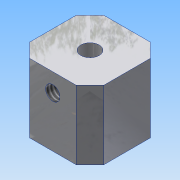
# Autodesk Inventor part: Drehmomentuebertraeger_V4_1
Saved by Autodesk Inventor 2015 (Build 190159000, 159)
## iProperties
Created: 2015-09-28
Part Number: Drehmomentuebertraeger_V4_1
Material: Aluminium 6061
Document SubType Name: Modeling
Designer: Johann
Density: 2.7 g/cm^3
Appearance: Aluminium - flach
Author: Johann
Autodesk Inventor part; units mm, degrees
ref_plane "YZ Plane" through (0, 0, 0) normal (1, 0, 0) x (0, 1, 0)
ref_plane "XZ Plane" through (0, 0, 0) normal (0, 1, 0) x (-1, 0, 0)
ref_plane "XY Plane" through (0, 0, 0) normal (0, 0, 1) x (1, 0, 0)
sketch "Skizze1" plane through (0, 0, 0) normal (0, 0, 1) x (1, 0, 0)
  line L0 (-4.05, -4.05) -> (4.05, -4.05)
  line L1 (4.05, -4.05) -> (4.05, 4.05)
  line L2 (4.05, 4.05) -> (-4.05, 4.05)
  line L3 (-4.05, 4.05) -> (-4.05, -4.05)
  line L4 (-4.05, -4.05) -> (4.05, 4.05) construction
  line L5 (4.05, -4.05) -> (-4.05, 4.05) construction
  point P0 (0, 0)
  dimension "d0" = 8.1
  constraints: 12 end point, 2 midpoint, 2 parallel, 2 perpendicular, 1 horizontal
  measures "d0" distance of L2.end L1.end
extrude "Extrusion1" add sketch "Skizze1" along normal blind 7.5
sketch "Skizze3" plane through (0, 0, 7.5) normal (0, 0, 1) x (1, 0, 0)
  point P0 (0, 0)
  point P1 (0, 0)
  constraints: 1 coincident
hole "Bohrung1" at (0, 0, 7.5) direction (0, 0, -1) diameter 2 end through all
sketch "Skizze4" plane through (-4.05, 4.05, 0) normal (0, 1, 0) x (1, 0, 0)
  line L0 (8.1, 0) -> (0, 0) construction
  line L1 (0, 0) -> (0, -7.5) construction
  line L2 (8.1, -7.5) -> (0, -7.5) construction
  line L3 (8.1, 0) -> (8.1, -7.5) construction
  line L4 (8.1, -7.5) -> (0, -7.5) projected
  line L5 (4.05, -7.5) -> (4.05, 0) construction
  point P0 (4.05, -5.5)
  dimension "d11" = 2
  constraints: 2 end point, 1 midpoint, 1 point on line, 1 vertical
  measures "d11" distance from line of L2 point (4.05, -5.5)
hole "Bohrung2" at (0, 4.05, 5.5) direction (0, -1, 0) diameter 1.567 end through all thread size "M2x0.4" class "6H" standard "ISO Metric profile"
chamfer "Fase1" distance 1.5 angle 45 4 edges at (-4.05, 4.05, 3.75) (4.05, 4.05, 3.75) (-4.05, -4.05, 3.75) (4.05, -4.05, 3.75)
